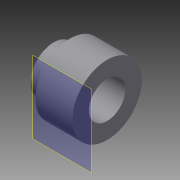
# Autodesk Inventor part: union pvc tubo
Saved by Autodesk Inventor 2013 (Build 170138000, 138)
## iProperties
Created: 2013-04-15
Part Number: union pvc tubo
Material: Generic
Document SubType Name: Modeling
Designer: Sebastian Saez
Density: 1 g/cm^3
Author: Sebastian Saez
Autodesk Inventor part; units mm, degrees
ref_plane "YZ Plane" through (0, 0, 0) normal (1, 0, 0) x (0, 1, 0)
ref_plane "XY Plane" through (0, 0, 0) normal (0, 0, 1) x (1, 0, 0)
sketch "Sketch1" plane through (0, 0, 0) normal (1, 0, 0) x (0, 1, 0)
  circle A0 centre (0, 0) radius 16.5
  circle A1 centre (0, 0) radius 19.5
  dimension "d0" = 33
  dimension "d1" = 3
  constraints: 2 centre point, 2 coincident
  measures "d0" diameter of A0
  measures "d1" radial gap between concentric circles of A1 A0
extrude "Extrusion1" add sketch "Sketch1" along normal blind 20.75 contours A0 | A1
sketch "Sketch2" plane through (0, 0, 0) normal (-1, 0, 0) x (0, 0, 1)
  circle A0 centre (0, 0) radius 19.5 projected
  circle A1 centre (0, 0) radius 16.5
  dimension "d4" = 33
  constraints: 1 centre point, 1 coincident
  measures "d4" diameter of A1
extrude "Extrusion2" cut sketch "Sketch2" against normal blind 25 contours A1
ref_plane "Work Plane2" through (0, -19.5, 0) normal (0, 1, 0) x (-1, 0, 0)
sketch "Sketch6" plane through (20.75, 0, 0) normal (1, 0, 0) x (0, 0, -1)
  circle A0 centre (0, 0) radius 10.25 projected
  circle A1 centre (0, 0) radius 19.5 projected
  circle A2 centre (0, 0) radius 13
  dimension "d14" = 26
  constraints: 1 centre point, 1 coincident
  measures "d14" diameter of A2
extrude "Extrusion5" add sketch "Sketch6" against normal blind 30 contours A2
sketch "Sketch7" plane through (20.75, 0, 0) normal (1, 0, 0) x (0, 0, -1)
  circle A0 centre (0, 0) radius 19.5 projected
  circle A1 centre (0, 0) radius 19.5
  circle A2 centre (0, 0) radius 16.5 projected
  circle A3 centre (0, 0) radius 10.25
  dimension "d23" = 20.5
  constraints: 2 centre point, 2 coincident, 1 concentric
  measures "d23" diameter of A3
extrude "Extrusion7" add sketch "Sketch7" against normal blind 2 contours A2
body "Solid1"
